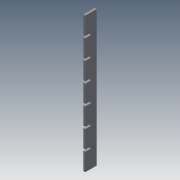
# Autodesk Inventor part: leg
Saved by Autodesk Inventor 2015 (Build 190159000, 159)
## iProperties
Created: 2014-09-01
Part Number: leg
Material: Generic
Document SubType Name: Modeling
Designer: shohei
Density: 1 g/cm^3
Appearance: Default
Author: shohei
Autodesk Inventor part; units mm, degrees
ref_plane "YZ Plane" through (0, 0, 0) normal (1, 0, 0) x (0, 1, 0)
ref_plane "XZ Plane" through (0, 0, 0) normal (0, 1, 0) x (-1, 0, 0)
ref_plane "XY Plane" through (0, 0, 0) normal (0, 0, 1) x (1, 0, 0)
sketch "Sketch1" plane through (0, 0, 0) normal (1, 0, 0) x (0, 1, 0)
  line L0 (0, 0) -> (50, 0)
  line L1 (50, 0) -> (50, 600)
  line L2 (50, 600) -> (0, 600)
  line L3 (0, 600) -> (0, 0)
  line L4 (0, 78) -> (25, 78)
  line L5 (25, 78) -> (25, 87)
  line L6 (25, 87) -> (0, 87)
  line L7 (0, 87) -> (0, 78)
  line L8 (0, 165) -> (25, 165)
  line L9 (25, 165) -> (25, 174)
  line L10 (25, 174) -> (0, 174)
  line L11 (0, 174) -> (0, 165)
  line L12 (0, 252) -> (25, 252)
  line L13 (25, 252) -> (25, 261)
  line L14 (25, 261) -> (0, 261)
  line L15 (0, 261) -> (0, 252)
  line L16 (0, 339) -> (25, 339)
  line L17 (25, 339) -> (25, 348)
  line L18 (25, 348) -> (0, 348)
  line L19 (0, 348) -> (0, 339)
  line L20 (0, 426) -> (25, 426)
  line L21 (25, 426) -> (25, 435)
  line L22 (25, 435) -> (0, 435)
  line L23 (0, 435) -> (0, 426)
  line L24 (0, 513) -> (25, 513)
  line L25 (25, 513) -> (25, 522)
  line L26 (25, 522) -> (0, 522)
  line L27 (0, 522) -> (0, 513)
  dimension "d0" = 50
  dimension "d1" = 600
  dimension "d4" = 9
  dimension "d5" = 25
  dimension "d6" = 78
  dimension "d7" = 9
  dimension "d8" = 25
  dimension "d9" = 9
  dimension "d10" = 25
  dimension "d11" = 9
  dimension "d12" = 25
  dimension "d13" = 9
  dimension "d14" = 25
  dimension "d15" = 9
  dimension "d16" = 25
  dimension "d17" = 78
  dimension "d18" = 78
  dimension "d19" = 78
  dimension "d20" = 78
  dimension "d21" = 78
  constraints: 56 end point, 14 parallel, 7 horizontal, 7 perpendicular, 1 point on line
  measures "d0" distance of L1.end L2.end
  measures "d1" distance of L0.end L1.end
  measures "d4" distance of L4.end L5.end
  measures "d5" distance of L4.start L4.end
  measures "d6" distance between parallel lines of L0 L4
  measures "d7" distance of L8.end L9.end
  measures "d8" distance of L8.start L8.end
  measures "d9" distance of L12.end L13.end
  measures "d10" distance of L12.start L12.end
  measures "d11" distance of L16.end L17.end
  measures "d12" distance of L16.start L16.end
  measures "d13" distance of L20.end L21.end
  measures "d14" distance of L20.start L20.end
  measures "d15" distance of L24.end L25.end
  measures "d16" distance of L24.start L24.end
  measures "d17" distance between parallel lines of L8 L6
  measures "d18" distance between parallel lines of L12 L10
  measures "d19" distance between parallel lines of L16 L14
  measures "d20" distance between parallel lines of L20 L18
  measures "d21" distance between parallel lines of L24 L22
extrude "Extrusion2" add sketch "Sketch1" along normal blind 9 contours L3 L4 L5 L6 L8 L9 L10 L12 L13 L14 L16 L17 L18 L20 L21 L22 L24 L25 L26 L2 L1 L0
equation "\"d17\" = d6"
equation "\"d18\" = d6"
equation "\"d19\" = d6"
equation "\"d20\" = d6"
equation "\"d21\" = d6"
body "Solid2"
